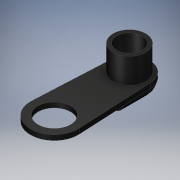
# Autodesk Inventor part: Absaugschuh
Saved by Autodesk Inventor 2019 (Build 230136000, 136)
## iProperties
Created: 2021-04-25
Part Number: Absaugschuh
Material: PET-Kunststoff
Document SubType Name: Modeling
Designer: Michael Sumper
Density: 1.541 g/cm^3
Appearance: PTFE
Author: Michael Sumper
Autodesk Inventor part; units mm, degrees
ref_plane "YZ Plane" through (0, 0, 0) normal (1, 0, 0) x (0, 1, 0)
ref_plane "XZ Plane" through (0, 0, 0) normal (0, 1, 0) x (-1, 0, 0)
sketch "Skizze1" plane through (0, 0, 0) normal (0, 1, 0) x (-1, 0, 0)
  circle A0 centre (0, 0) radius 32.5
  circle A1 centre (0, 0) radius 47.5
  line L0 (0, 0) -> (0, -150) construction
  circle A2 centre (0, -150) radius 25
  circle A3 centre (0, -150) radius 40
  line L1 (47.4406, -2.375) -> (39.95, -152)
  line L2 (-47.4406, -2.375) -> (-39.95, -152)
  dimension "d0" = 65
  dimension "d1" = 15
  dimension "d2" = 150
  dimension "d3" = 50
  dimension "d4" = 15
  constraints: 6 end point, 4 centre point, 4 point on circle, 4 tangent, 2 coincident, 1 vertical
  measures "d0" diameter of A0
  measures "d1" radial gap between concentric circles of A0 A1
  measures "d2" distance of L0.start L0.end
  measures "d3" diameter of A2
  measures "d4" radial gap between concentric circles of A2 A3
extrude "Extrusion1" add sketch "Skizze1" along normal blind 10
sketch "Skizze2" plane through (0, 10, 0) normal (0, 1, 0) x (1, 0, 0)
  circle A0 centre (0, 150) radius 25 projected
  circle A1 centre (0, 150) radius 32.5
  point P0 (0, 0)
  dimension "d7" = 7.5
  constraints: 1 centre point
  measures "d7" radial gap between concentric circles of A0 A1
extrude "Extrusion2" add sketch "Skizze2" along normal blind 50
ref_plane "Arbeitsebene1" through (0, 0, -190) normal (-1, 0, 0) x (0, -1, 0)
sketch "Skizze3" plane through (0, 0, -190) normal (-1, 0, 0) x (0, -1, 0)
  line L0 (0, 38) -> (0, 0) projected
  line L1 (0, 10.9925) -> (10.9925, 10.9925) construction
  line L2 (0, 10.9925) -> (0, 0) construction
  line L3 (0, 0) -> (0, 3)
  line L4 (0, 38) -> (-10, 38) construction
  line L5 (0, 38) -> (16.612, 38) construction
  arc A0 (0, 10.9925) -> (10.4174, 17.007) centre (0, 23.0214) ccw
  line L6 (0, 23.0214) -> (12.0289, 23.0214) construction
  line L7 (0, 23.0214) -> (0, 10.9925) construction
  line L8 (-10.9478, 2.8205) -> (-10.9478, 33.9693) construction
  line L9 (-10.9478, 33.9693) -> (20.2009, 33.9693) construction
  line L10 (22.6543, 38) -> (21.7274, 15.548)
  arc A1 (0, 0.0447) -> (21.7274, 15.548) centre (0, 23.0214) ccw
  line L11 (0, 10.9925) -> (0, 3)
  line L12 (10.4174, 17.007) -> (22.6543, 38)
  point P0 (0, 190)
  dimension "d12" = 90
  constraints: 22 end point, 5 point on line, 4 point on circle, 2 centre point, 1 collinear, 1 horizontal, 5 other
  measures "d12" angle of L7 L6
revolve "Umdrehung1" add sketch "Skizze3" angle 180 mid plane about axis through (0, 0, -152) along (0, -1, 0)
sketch "Skizze4" plane through (-37.9553, 0, -152) normal (0, 0, 1) x (1, 0, 0)
  line L0 (64.9628, 0) -> (75.9106, 0) projected
  arc A0 (58.9484, -10.4174) -> (64.9628, 0) centre (52.9339, 0) ccw projected
  line L1 (58.9484, -10.4174) -> (37.9553, -22.6543) projected
  line L2 (37.9553, -22.6543) -> (60.4073, -21.7274) projected
  arc A1 (60.4073, -21.7274) -> (75.9106, 0) centre (52.9339, 0) ccw projected
  line L3 (0, 0) -> (10.9478, 0) projected
  arc A2 (0, 0) -> (15.5034, -21.7274) centre (22.9768, 0) ccw projected
  line L4 (15.5034, -21.7274) -> (37.9553, -22.6543) projected
  line L5 (37.9553, -22.6543) -> (16.9623, -10.4174) projected
  arc A3 (10.9478, 0) -> (16.9623, -10.4174) centre (22.9768, 0) ccw projected
  point P0 (37.9553, 0)
extrude "Extrusion3" add sketch "Skizze4" along normal blind 50
sketch "Skizze5" plane through (-37.9553, 0, -102) normal (0, 0, 1) x (1, 0, 0)
  line L0 (22.9553, -21.6543) -> (52.9553, -21.6543)
  line L1 (52.9553, -21.6543) -> (52.9553, -23.6543)
  line L2 (52.9553, -23.6543) -> (22.9553, -23.6543)
  line L3 (22.9553, -23.6543) -> (22.9553, -21.6543)
  line L4 (37.9553, -22.6543) -> (16.9623, -10.4174) projected
  line L5 (22.9553, -21.6543) -> (52.9553, -23.6543) construction
  line L6 (52.9553, -21.6543) -> (22.9553, -23.6543) construction
  point P0 (37.9553, 0)
  dimension "d16" = 30
  dimension "d17" = 2
  constraints: 12 end point, 2 midpoint, 2 parallel, 1 horizontal, 1 perpendicular
  measures "d16" distance of L1.end L2.end
  measures "d17" distance of L0.end L1.end
extrude "Extrusion4" add sketch "Skizze5" against normal blind 60
